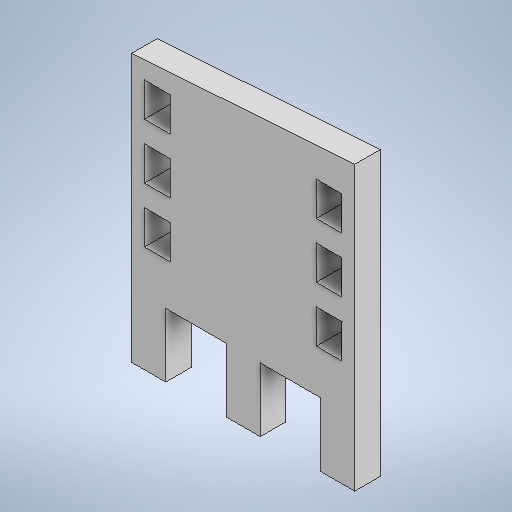
# Autodesk Inventor part: sort support V2 wall 1
Saved by Autodesk Inventor 2025.3 (Build 293356000, 356)
## iProperties
Created: 2026-04-30
Part Number: sort support V2 wall 1
Material: Generic
Document SubType Name: Modeling
Designer: kamal
Density: 1 g/cm^3
Appearance: Default
Author: kamal
Autodesk Inventor part; units mm, degrees
ref_plane "YZ Plane" through (0, 0, 0) normal (1, 0, 0) x (0, 1, 0)
ref_plane "XZ Plane" through (0, 0, 0) normal (0, 1, 0) x (-1, 0, 0)
ref_plane "XY Plane" through (0, 0, 0) normal (0, 0, 1) x (1, 0, 0)
sketch "Sketch1" plane through (0, 0, 0) normal (0, 0, 1) x (1, 0, 0)
  line L0 (0, 0) -> (0, 47.913)
  line L1 (0, 0) -> (52.4, 0)
  line L2 (52.4, 0) -> (52.4, 51.52)
  line L3 (52.4, 51.52) -> (0, 47.913)
  line L4 (3, 44) -> (9, 44)
  line L5 (9, 44) -> (9, 36)
  line L6 (9, 36) -> (3, 36)
  line L7 (3, 36) -> (3, 44)
  line L8 (3, 31) -> (9, 31)
  line L9 (9, 31) -> (9, 23)
  line L10 (9, 23) -> (3, 23)
  line L11 (3, 23) -> (3, 31)
  line L12 (3, 18) -> (9, 18)
  line L13 (9, 18) -> (9, 10)
  line L14 (9, 10) -> (3, 10)
  line L15 (3, 10) -> (3, 18)
  line L16 (26.2, 0) -> (26.2, 49.7165) construction
  line L17 (49.4, 44) -> (43.4, 44)
  line L18 (43.4, 44) -> (43.4, 36)
  line L19 (43.4, 36) -> (49.4, 36)
  line L20 (49.4, 36) -> (49.4, 44)
  line L21 (49.4, 31) -> (43.4, 31)
  line L22 (43.4, 31) -> (43.4, 23)
  line L23 (43.4, 23) -> (49.4, 23)
  line L24 (49.4, 23) -> (49.4, 31)
  line L25 (49.4, 18) -> (43.4, 18)
  line L26 (43.4, 18) -> (43.4, 10)
  line L27 (43.4, 10) -> (49.4, 10)
  line L28 (49.4, 10) -> (49.4, 18)
  line L29 (0, 0) -> (0, -15)
  line L30 (0, -15) -> (8, -15)
  line L31 (8, -15) -> (8, 0)
  line L32 (52.4, 0) -> (52.4, -15)
  line L33 (52.4, -15) -> (44.4, -15)
  line L34 (44.4, -15) -> (44.4, 0)
  line L35 (22.2, 0) -> (30.2, 0)
  line L36 (30.2, 0) -> (30.2, -15)
  line L37 (30.2, -15) -> (22.2, -15)
  line L38 (22.2, -15) -> (22.2, 0)
  point P0 (3, 14)
  point P1 (3, 27)
  point P2 (3, 40)
  point P3 (6, 10)
  point P4 (6, 23)
  point P5 (6, 18)
  point P6 (6, 36)
  point P7 (6, 31)
  dimension "d0" = 47.913
  dimension "d1" = 52.4
  dimension "d2" = 51.52
  dimension "d3" = 6
  dimension "d4" = 8
  dimension "d5" = 6
  dimension "d6" = 8
  dimension "d7" = 6
  dimension "d8" = 8
  dimension "d9" = 3
  dimension "d10" = 3
  dimension "d11" = 3
  dimension "d12" = 10
  dimension "d13" = 5
  dimension "d14" = 5
  dimension "d17" = 15
  dimension "d18" = 8
  dimension "d19" = 8
  dimension "d20" = 15
  dimension "d21" = 8
  dimension "d22" = 15
  dimension "d24" = 14.2
  constraints: 78 end point, 12 symmetric about line, 10 midpoint, 9 parallel, 7 perpendicular, 5 horizontal, 5 point on line, 3 vertical
  measures "d0" distance of L0.start L0.end
  measures "d1" distance of L0.start L1.end
  measures "d2" distance of L1.end L2.end
  measures "d3" distance of L5.end L6.end
  measures "d4" distance of L4.end L5.end
  measures "d5" distance of L9.end L10.end
  measures "d6" distance of L8.end L9.end
  measures "d7" distance of L13.end L14.end
  measures "d8" distance of L12.end L13.end
  measures "d9" distance from line of L0 point (3, 14)
  measures "d10" distance from line of L0 point (3, 27)
  measures "d11" distance from line of point (3, 40) L0
  measures "d12" distance from line of point (6, 10) L1
  measures "d13" distance of point (6, 23) point (6, 18)
  measures "d14" distance of point (6, 36) point (6, 31)
  measures "d17" distance of L0.start L29.end
  measures "d18" distance of L29.end L30.end
  measures "d19" distance between parallel lines of L34 L2
  measures "d20" distance of L1.end L32.end
  measures "d21" distance of L36.end L37.end
  measures "d22" distance of L35.end L36.end
  measures "d24" distance between parallel lines of L31 L38
extrude "Extrusion1" add sketch "Sketch1" along normal blind 6 contours L0 L3 L2 L1
extrude "Extrusion2" add sketch "Sketch1" along normal blind 6 contours L1 L31 L30 L29 | L1 L36 L37 L38 | L32 L33 L34 L1
body "Solid1"
